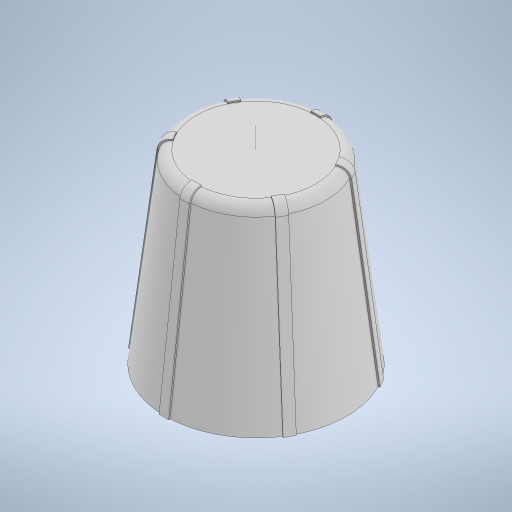
# Autodesk Inventor part: Drehencoder
Saved by Autodesk Inventor 2023.1 (Build 271208000, 208)
## iProperties
Created: 2023-04-27
Part Number: Drehencoder
Material: Generisch
Document SubType Name: Sheet Metal
Designer: marco
Density: 1 g/cm^3
Sheet Metal Rule: Standard_mm
Appearance: Vorgabe
Author: marco
Autodesk Inventor part; units mm, degrees
ref_plane "YZ Plane" through (0, 0, 0) normal (1, 0, 0) x (0, 1, 0)
ref_plane "XZ Plane" through (0, 0, 0) normal (0, 1, 0) x (-1, 0, 0)
ref_plane "XY Plane" through (0, 0, 0) normal (0, 0, 1) x (1, 0, 0)
sketch "Skizze1" plane through (0, 0, 0) normal (1, 0, 0) x (0, 1, 0)
  line L0 (0, 0) -> (12, 0)
  line L1 (12, 0) -> (12, -3.1)
  line L2 (12, -3.1) -> (0, -3.1)
  line L3 (0, -3.1) -> (0, -6.6)
  line L4 (12, 0) -> (13.5, 0)
  line L5 (13.5, 0) -> (13.5, -5)
  line L6 (13.5, -5) -> (0, -6.6)
  dimension "d0" = 12
  dimension "d1" = 3.1
  dimension "d2" = 3.5
  dimension "d3" = 1.5
  dimension "d4" = 5
  constraints: 14 end point, 4 perpendicular, 2 horizontal
  measures "d0" distance of L0.start L0.end
  measures "d1" distance of L0.end L1.end
  measures "d2" distance of L2.end L3.end
  measures "d3" distance of L0.end L4.end
  measures "d4" distance of L4.end L5.end
revolve "Umdrehung1" add sketch "Skizze1" angle 360 about axis through (0, 0, 0) along (0, 1, 0)
fillet "Rundung1" radius 0.75 1 edges at (0, 13.5, 5)
sketch "Skizze2" plane through (0, 0, 0) normal (1, 0, 0) x (0, 1, 0)
  line L0 (13.5, 4.3336) -> (13.5, -4.3336) projected
  line L1 (13.5, 0) -> (13.6, 0)
  line L2 (13.5, 0) -> (13.6, 0) construction
  line L3 (13.6, 0) -> (13.6, 4.3336)
  line L4 (13.6, 4.3336) -> (12.8383, 4.3336)
  line L5 (12.8383, -5.0784) -> (12.8383, 5.0784) projected
  line L6 (0, 6.6) -> (12.8383, 5.0784) projected
  line L7 (0, 6.6) -> (0, 6.7)
  line L8 (0, 6.6) -> (0.1, 6.6) construction
  arc A0 (13.6, 4.3336) -> (12.8388, 5.1897) centre (12.7381, 4.3336) ccw
  line L9 (12.8388, 5.1897) -> (0, 6.7)
  point P0 (0, 0)
  dimension "d7" = 0.1
  dimension "d8" = 0
  dimension "d9" = 0.1
  dimension "d10" = 90
  constraints: 14 end point, 3 perpendicular, 2 equal length, 2 horizontal, 2 point on circle, 2 point on line, 1 centre point, 1 midpoint, 1 tangent, 1 vertical
  measures "d7" distance of L1.start L1.end
  measures "d8" distance between parallel lines of L1 L2
  measures "d9" distance of L7.start L7.end
  measures "d10" angle of L8 L7
extrude "Extrusion1" add sketch "Skizze2" along normal mid plane 0.7 contours L4 L5 L6 L7 L9 A0
pattern_circular "Runde Anordnung1" count 6 over 360 about axis through (0, 13.5, 0) along (0, -1, 0) of "Extrusion1"
thicken "Verdickung1" operation cut thickness 0.1 both sides no extend neighbours no toward (0.1604113, 0, -0.9870503) faces at (0.4973, 8, -3.0599)
sketch "Skizze3" plane through (0, 12, 0) normal (0, -1, 0) x (1, 0, 0)
  circle A0 centre (0, 0) radius 3.2 projected
  line L0 (-1.4, 2.8775) -> (-1.4, -2.8775)
  arc A1 (-1.4, 2.8775) -> (-1.4, -2.8775) centre (0, 0) ccw
  dimension "d18" = 4.6
  constraints: 4 point on circle, 2 end point, 1 centre point, 1 coincident, 1 vertical
extrude "Extrusion2" add sketch "Skizze3" along normal blind 8 contours L0 A0 picked at (-1.6215, -0.815)
thicken "Verdickung2" operation cut thickness 0.2 both sides no extend neighbours no toward (-1, 0, 0) faces at (-1.4, 9.3333, -0.9592)
equation "\"Biegeradius\" = Stärke"
equation "\"BreiteBiegungsfreistellung\" = Stärke"
equation "\"TiefeBiegungsfreistellung\" = 0.5 * Stärke"
equation "\"GrößeEckenfreistellung\" = 4 * Stärke"
equation "\"MinimalRest\" = 2 * Stärke"
equation "\"Übergangsradius\" = Biegeradius"
equation "\"JacobiRadiusGröße\" = Biegeradius"
equation "\"Abstandsgröße\" = Stärke"
equation "\"Stärke\" = 0.5"
